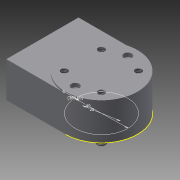
# Autodesk Inventor part: CFS055CA501U
Saved by Autodesk Inventor 2013 (Build 170138000, 138)
## iProperties
Created: 2013-01-30
Part Number: CFS055CA501U
Material: Generic
Document SubType Name: Modeling
Designer: Mahisorn
Density: 1 g/cm^3
Author: Mahisorn
Autodesk Inventor part; units mm, degrees
ref_plane "YZ Plane" through (0, 0, 0) normal (1, 0, 0) x (0, 1, 0)
ref_plane "XZ Plane" through (0, 0, 0) normal (0, 1, 0) x (-1, 0, 0)
ref_plane "XY Plane" through (0, 0, 0) normal (0, 0, 1) x (1, 0, 0)
sketch "Sketch1" plane through (0, 0, 0) normal (0, 1, 0) x (-1, 0, 0)
  circle A0 centre (0, 0) radius 27.5
  point P0 (20, 0)
  point P1 (14.1421, 14.1421)
  point P2 (0, 20)
  point P3 (-14.1421, 14.1421)
  point P4 (-20, 0)
  point P5 (-14.1421, -14.1421)
  point P6 (0, -20)
  point P7 (14.1421, -14.1421)
  dimension "d0" = 55
  dimension "d19" = 20
  dimension "d22" = 360
  constraints: 1 centre point, 1 coincident, 9 other
  measures "d0" diameter of A0
  measures "d19" distance of point (0, 0) point (20, 0)
extrude "Extrusion1" add sketch "Sketch1" against normal blind 28
sketch "Sketch2" plane through (0, -28, 0) normal (0, -1, 0) x (1, 0, 0)
  circle A0 centre (0, 0) radius 27.5 projected
  line L0 (0, 27.5) -> (45, 27.5)
  line L1 (45, 27.5) -> (45, -27.5)
  line L2 (45, -27.5) -> (0, -27.5)
  dimension "d15" = 45
  dimension "d16" = 55
  constraints: 6 end point, 2 point on circle, 2 tangent, 1 horizontal, 1 perpendicular
  measures "d15" distance of L0.start L0.end
  measures "d16" distance of L0.end L1.end
extrude "Extrusion2" add sketch "Sketch2" against normal blind 27 contours A0 L0 L1 L2
hole "Hole1" at (0, 0, 20) at (0, 0, -20) direction (0, -1, 0) diameter 6 depth 3 tip angle 118
hole "Hole2" at (-14.1421, 0, 14.1421) at (14.1421, 0, 14.1421) at (14.1421, 0, -14.1421) at (-14.1421, 0, -14.1421) direction (0, -1, 0) diameter 4.917 depth 8 tip angle 118 thread size "M6x1" class "6H" standard "ANSI Metric M Profile"
sketch "Sketch3" plane through (0, -28, 0) normal (0, -1, 0) x (1, 0, 0)
  arc A0 (0, 27.5) -> (0, -27.5) centre (0, 0) ccw projected
  circle A1 centre (0, 0) radius 12.5
  circle A2 centre (0, 0) radius 20
  circle A3 centre (20, 0) radius 3
  circle A4 centre (14.1421, 14.1421) radius 3
  circle A5 centre (0, 20) radius 3
  circle A6 centre (-14.1421, 14.1421) radius 3
  circle A7 centre (-20, 0) radius 3
  circle A8 centre (-14.1421, -14.1421) radius 3
  circle A9 centre (0, -20) radius 3
  circle A10 centre (14.1421, -14.1421) radius 3
  dimension "d44" = 40
  dimension "d38" = 25
  dimension "d45" = 6
  dimension "d48" = 360
  constraints: 9 centre point, 2 coincident, 1 horizontal alignment, 19 other
  measures "d38" diameter of A1
  measures "d45" diameter of A3
extrude "Extrusion3" add sketch "Sketch3" along normal blind 3 contours A1
chamfer "Chamfer1" distance 0.5 angle 45 1 edges at (-12.5, -31, 0)
extrude "Extrusion4" add sketch "Sketch3" along normal blind 6 contours A4 A2 | A2 A4 | A10 A2 | A2 A10 | A6 A2 | A2 A6 | A8 A2 | A2 A8
thread "Thread1" size "M6x1" class "6g" standard "ANSI Metric M Profile" full length
thread "Thread2" size "M6x1" class "6g" standard "ANSI Metric M Profile" full length
thread "Thread3" size "M6x1" class "6g" standard "ANSI Metric M Profile" full length
thread "Thread4" size "M6x1" class "6g" standard "ANSI Metric M Profile" full length
chamfer "Chamfer2" distance 0.5 angle 45 1 edges at (-17.1421, -34, -14.1421)
chamfer "Chamfer3" distance 0.5 angle 45 1 edges at (-17.1421, -34, 14.1421)
chamfer "Chamfer4" distance 0.5 angle 45 1 edges at (11.1421, -34, 14.1421)
chamfer "Chamfer5" distance 0.5 angle 45 1 edges at (11.1421, -34, -14.1421)
hole "Hole3" at (0, -28, 20) at (0, -28, -20) direction (0, 1, 0) diameter 6 depth 3 tip angle 118
body "Solid1"
